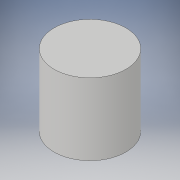
# Autodesk Inventor part: cargo
Saved by Autodesk Inventor 2018 (Build 220112000, 112)
## iProperties
Created: 2018-04-22
Part Number: cargo
Material: Generic
Document SubType Name: Modeling
Designer: atbin
Density: 0.231958 g/cm^3
Appearance: Default
Mass: 1.45744e+06 g
Surface Area: 188496 cm^2
Volume: 6.28319e+06 cm^3
Author: atbin
Autodesk Inventor part; units mm, degrees
ref_plane "YZ Plane" through (0, 0, 0) normal (1, 0, 0) x (0, 1, 0)
ref_plane "XZ Plane" through (0, 0, 0) normal (0, 1, 0) x (-1, 0, 0)
ref_plane "XY Plane" through (0, 0, 0) normal (0, 0, 1) x (1, 0, 0)
sketch "Sketch1" plane through (0, 0, 0) normal (0, 0, 1) x (1, 0, 0)
  line L0 (0, 1000) -> (1000, 1000)
  line L1 (1000, 1000) -> (1000, -1000)
  line L2 (1000, -1000) -> (0, -1000)
  line L3 (0, -1000) -> (0, 1000)
  line L4 (-200, 0) -> (1200, 0) projected
  point P0 (0, 0)
  dimension "d0" = 2000
  dimension "d1" = 1000
  dimension "d2" = 1000
  constraints: 8 end point, 2 parallel, 1 horizontal, 1 perpendicular
  measures "d0" distance of L2.end L0.start
  measures "d1" distance between parallel lines of L4 L2
  measures "d2" distance between parallel lines of L1 L3
revolve "Revolution1" add sketch "Sketch1" angle 360 about axis through (0, -1000, 0) along (0, 1, 0)
body "Solid1"
